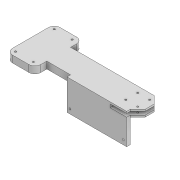
# Autodesk Inventor part: RobotBaseMotorExt
Saved by Autodesk Inventor 2022 (Build 260153000, 153)
## iProperties
Created: 2022-10-20
Part Number: RobotBaseMotorExt
Material: Generic
Document SubType Name: Modeling
Designer: MVeszpremi
Density: 1 g/cm^3
Appearance: Default
Author: MVeszpremi
Autodesk Inventor part; units mm, degrees
ref_plane "YZ Plane" through (0, 0, 0) normal (1, 0, 0) x (0, 1, 0)
ref_plane "XZ Plane" through (0, 0, 0) normal (0, 1, 0) x (-1, 0, 0)
sketch "Sketch1" plane through (0, 0, 0) normal (0, 1, 0) x (-1, 0, 0)
  line L0 (0, 0) -> (200, 0)
  line L1 (200, 0) -> (200, -80)
  line L2 (200, -80) -> (0, -80)
  line L3 (0, -80) -> (0, 0)
  line L4 (10, -30) -> (30, -30)
  line L5 (30, -30) -> (30, -50)
  line L6 (30, -50) -> (10, -50)
  line L7 (10, -50) -> (10, -30)
  circle A0 centre (10, -30) radius 1.5
  circle A1 centre (30, -50) radius 1.5
  circle A2 centre (30, -30) radius 1.5
  circle A3 centre (10, -50) radius 1.5
  line L8 (192.5, -7.5) -> (162.5, -7.5)
  line L9 (162.5, -7.5) -> (162.5, -72.5)
  line L10 (162.5, -72.5) -> (192.5, -72.5)
  line L11 (192.5, -72.5) -> (192.5, -7.5)
  circle A4 centre (192.5, -7.5) radius 1.5
  circle A5 centre (192.5, -72.5) radius 1.5
  circle A6 centre (162.5, -72.5) radius 1.5
  circle A7 centre (162.5, -7.5) radius 1.5
  line L12 (200, 0) -> (152.5, 0)
  line L13 (152.5, 0) -> (152.5, -80)
  line L14 (152.5, -80) -> (200, -80)
  line L15 (200, -80) -> (200, 0)
  line L16 (152.5, -20) -> (0, -20)
  line L17 (0, -20) -> (0, -60)
  line L18 (0, -60) -> (152.5, -60)
  line L19 (152.5, -60) -> (152.5, -20)
  line L20 (40, -20) -> (40, -60)
  point P0 (191, -7.5)
  point P1 (192.5, -9)
  point P2 (192.5, -71)
  point P3 (191, -72.5)
  point P4 (164, -72.5)
  point P5 (162.5, -71)
  point P6 (164, -7.5)
  point P7 (162.5, -9)
  point P8 (152.5, 0)
  point P9 (0, -20)
  dimension "d0" = 200
  dimension "d1" = 80
  dimension "d2" = 20
  dimension "d3" = 20
  dimension "d4" = 30
  dimension "d5" = 10
  dimension "d6" = 3
  dimension "d7" = 3
  dimension "d8" = 3
  dimension "d9" = 3
  dimension "d10" = 65
  dimension "d11" = 30
  dimension "d12" = 7.5
  dimension "d13" = 7.5
  dimension "d14" = 3
  dimension "d15" = 3
  dimension "d16" = 3
  dimension "d17" = 3
  dimension "d18" = 20
  dimension "d19" = 20
  dimension "d20" = 10
  dimension "d23" = 40
  constraints: 42 end point, 10 parallel, 8 centre point, 8 coincident, 6 perpendicular, 5 horizontal, 5 point on line
  measures "d0" distance of L1.end L2.end
  measures "d1" distance of L0.end L1.end
  measures "d2" distance of L4.start L4.end
  measures "d3" distance of L4.end L5.end
  measures "d4" distance between parallel lines of L0 L4
  measures "d5" distance between parallel lines of L3 L7
  measures "d6" diameter of A2
  measures "d7" diameter of A1
  measures "d8" diameter of A3
  measures "d9" diameter of A0
  measures "d10" distance of L10.end L8.start
  measures "d11" distance of L8.start L8.end
  measures "d12" distance between parallel lines of L0 L8
  measures "d13" distance between parallel lines of L1 L11
  measures "d14" diameter of A4
  measures "d15" diameter of A7
  measures "d16" diameter of A6
  measures "d17" diameter of A5
  measures "d18" distance between parallel lines of L0 L16
  measures "d19" distance between parallel lines of L2 L18
  measures "d20" distance between parallel lines of L9 L19
  measures "d23" distance between parallel lines of L17 L20
extrude "Extrusion1" add sketch "Sketch1" along normal blind 3 contours L0 L1 L2 L13 | L16 L20 L18 L3 | L13 L18 L20 L16 | L4 A2 L5 A1 L6 A3 L7 A0 | L8 A4 L11 A5 L10 A6 L9 A7
extrude "Extrusion2" add sketch "Sketch1" against normal blind 5.5 contours L0 L1 L2 L13 | L13 L18 L20 L16 | L8 A4 L11 A5 L10 A6 L9 A7
ref_plane "Work Plane1" through (0, -2.75, 0) normal (0, -1, 0) x (1, 0, 0)
mirror "Mirror1" about plane through (0, -2.75, 0) normal (0, -1, 0) of "Extrusion1"
chamfer "Chamfer1" distance 12.5 angle 45 4 edges at (0, 1.5, -20) (0, -7, -20) (0, -7, -60) (0, 1.5, -60)
sketch "Sketch3" plane through (-152.5, -8.5, -20) normal (0, 0, 1) x (1, 0, 0)
  line L0 (152.5, 11.5) -> (0, 11.5) projected
  line L1 (140, 11.5) -> (40, 11.5)
  line L2 (40, 11.5) -> (40, -40)
  line L3 (40, -40) -> (140, -40)
  line L4 (140, -40) -> (140, 11.5)
  line L5 (112.5, 8.5) -> (112.5, 3) projected
  line L6 (112.5, 3) -> (140, 3) projected
  line L7 (112.5, 8.5) -> (112.5, 3) projected
  line L8 (112.5, 8.5) -> (140, 8.5) projected
  line L9 (0, 11.5) -> (140, 11.5) projected
  line L10 (0, 0) -> (0, 11.5) projected
  line L11 (0, 0) -> (140, 0) projected
  line L12 (0, 0) -> (140, 0) projected
  line L13 (122.5, 0) -> (122.5, 11.5)
  line L14 (0, 11.5) -> (152.5, 11.5) projected
  line L15 (140, -40) -> (140, -32.5)
  circle A0 centre (134.5, -32.5) radius 1.5
  line L16 (140, -32.5) -> (40, -32.5)
  circle A1 centre (45, -32.5) radius 1.5
  line L17 (140, 3) -> (140, 0) projected
  line L18 (140, 11.5) -> (140, 8.5) projected
  point P0 (152.5, 8.5)
  point P1 (147.5, 11.5)
  point P2 (140, 3)
  point P3 (140, 8.5)
  point P4 (40, 11.5)
  dimension "d30" = 100
  dimension "d32" = 7.5
  dimension "d33" = 3
  dimension "d34" = 3
  dimension "d35" = 89.5
  dimension "d36" = 5
  dimension "d40" = 40
  constraints: 14 end point, 6 point on line, 3 perpendicular, 2 centre point, 2 parallel, 1 horizontal
  measures "d30" distance of L2.end L3.end
  measures "d32" distance of L3.end L15.end
  measures "d33" diameter of A0
  measures "d34" diameter of A1
  measures "d35" distance of A1.centre A0.centre
  measures "d36" distance from line of L2 A1.centre
  measures "d40" distance between parallel lines of L3 L11
extrude "Extrusion3" add sketch "Sketch3" along normal blind 6 contours L4 L8 L13 L0 | L13 L8 L5 L6 L11 L2 L0 | L4 L11 L13 L6 | L11 L4 L16 A0 A1 L2 | L16 A1 A0 L4 L3 L2
sketch "Sketch4" plane through (-152.5, -8.5, -20) normal (0, 0, -1) x (-1, 0, 0)
  line L0 (-40, 11.5) -> (-40, -40) projected
  line L1 (-40, 0) -> (-140, 0)
  line L2 (-140, 0) -> (-140, -6)
  line L3 (-140, -6) -> (-40, -6)
  line L4 (-40, -6) -> (-40, 0)
  line L5 (-140, -40) -> (-140, 0) projected
  line L6 (-90, -6) -> (-90, 0)
  line L7 (-140, 0) -> (0, 0) projected
  point P0 (-152.5, 8.5)
  point P1 (-162.5, 0)
  dimension "d39" = 6
  constraints: 10 end point, 2 parallel, 2 perpendicular, 2 point on line, 1 horizontal, 1 midpoint
  measures "d39" distance between parallel lines of L1 L3
extrude "Extrusion4" add sketch "Sketch4" along normal blind 30 contours L0 L3 L6 L1
fillet "Fillet2" radius 10 4 edges at (-200, -2.75, -80) (-152.5, -2.75, -80) (-152.5, -2.75, 0) (-200, -2.75, 0)
body "Solid1"
